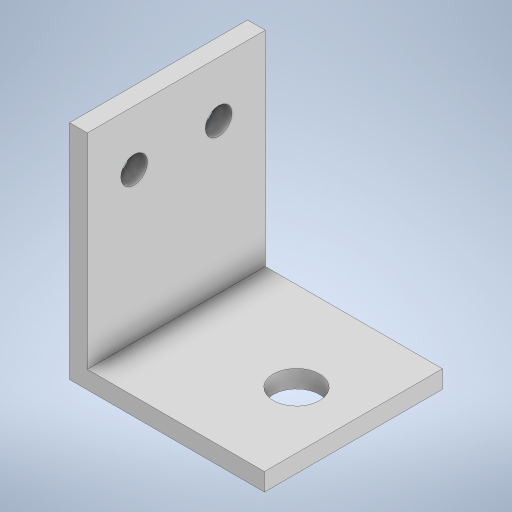
# Autodesk Inventor part: LimitSwitch Center Gantry Mount
Saved by Autodesk Inventor 2023.2 (Build 272271030, 271C)
## iProperties
Created: 2023-05-02
Part Number: LimitSwitch Center Gantry Mount
Material: Generic
Document SubType Name: Modeling
Designer: chase
Density: 1 g/cm^3
Appearance: Default
Author: chase
Autodesk Inventor part; units mm, degrees
ref_plane "YZ Plane" through (0, 0, 0) normal (1, 0, 0) x (0, 1, 0)
ref_plane "XZ Plane" through (0, 0, 0) normal (0, 1, 0) x (-1, 0, 0)
ref_plane "XY Plane" through (0, 0, 0) normal (0, 0, 1) x (1, 0, 0)
sketch "Sketch1" plane through (0, 0, 0) normal (0, 0, 1) x (1, 0, 0)
  line L0 (0, 0) -> (21.9, 0)
  line L1 (21.9, 0) -> (21.9, 25)
  line L2 (21.9, 25) -> (0, 25)
  line L3 (0, 25) -> (0, 0)
  line L4 (21.9, 25) -> (2, 25)
  line L5 (2, 25) -> (2, 2)
  line L6 (2, 2) -> (21.9, 2)
  line L7 (21.9, 2) -> (21.9, 25)
  point P0 (21.9, 2)
  dimension "d0" = 21.9
  dimension "d1" = 25
  dimension "d2" = 2
  dimension "d3" = 2
  constraints: 16 end point, 4 parallel, 2 horizontal, 2 perpendicular
  measures "d0" distance of L2.end L1.end
  measures "d1" distance of L1.end L0.end
  measures "d2" distance between parallel lines of L3 L5
  measures "d3" distance between parallel lines of L0 L6
extrude "Extrusion1" add sketch "Sketch1" against normal blind 20 contours L3 L2 L5 L6 L1 L0
sketch "Sketch2" plane through (0, 0, 0) normal (-1, 0, 0) x (0, 0, 1)
  line L0 (-20, 2) -> (-20, 0) projected
  line L1 (-20, 0) -> (-20, 18.8)
  line L2 (-20, 18.8) -> (0, 18.8)
  line L3 (0, 25) -> (0, 0) projected
  circle A0 centre (-14.75, 18.8) radius 1.5
  circle A1 centre (-5.25, 18.8) radius 1.5
  dimension "d6" = 18.8
  dimension "d7" = 3
  dimension "d8" = 3
  dimension "d9" = 9.5
  dimension "d10" = 5.25
  constraints: 4 end point, 3 point on line, 2 centre point, 1 collinear, 1 perpendicular
  measures "d6" distance of L0.end L1.end
  measures "d7" diameter of A0
  measures "d8" diameter of A1
  measures "d9" distance of A0.centre A1.centre
  measures "d10" distance from line of L3 A1.centre
extrude "Extrusion2" cut sketch "Sketch2" against normal through all
sketch "Sketch4" plane through (2, 2, 0) normal (0, 1, 0) x (1, 0, 0)
  line L0 (0, 0) -> (0, 20) projected
  line L1 (0, 10) -> (13.5, 10)
  circle A0 centre (13.5, 10) radius 2.6
  point P0 (-2, 0)
  dimension "d13" = 13.5
  dimension "d14" = 5.2
  constraints: 2 end point, 1 centre point, 1 coincident, 1 horizontal, 1 midpoint
  measures "d13" distance of L1.start L1.end
  measures "d14" diameter of A0
extrude "Extrusion3" cut sketch "Sketch4" against normal through all
body "Solid1"
